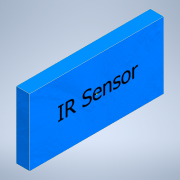
# Autodesk Inventor part: IR Sensor
Saved by Autodesk Inventor 2022.2 (Build 262287000, 287)
## iProperties
Created: 2022-02-24
Part Number: IR Sensor
Material: PVC-Piping
Document SubType Name: Modeling
Designer: PRASHANTH
Density: 1.4 g/cm^3
Appearance: Weld - Brass
Author: PRASHANTH
Autodesk Inventor part; units mm, degrees
ref_plane "YZ Plane" through (0, 0, 0) normal (1, 0, 0) x (0, 1, 0)
ref_plane "XZ Plane" through (0, 0, 0) normal (0, 1, 0) x (-1, 0, 0)
ref_plane "XY Plane" through (0, 0, 0) normal (0, 0, 1) x (1, 0, 0)
sketch "Sketch1" plane through (0, 0, 0) normal (1, 0, 0) x (0, 1, 0)
  line L0 (-7.5, 15) -> (7.5, 15)
  line L1 (7.5, 15) -> (7.5, -15)
  line L2 (7.5, -15) -> (-7.5, -15)
  line L3 (-7.5, -15) -> (-7.5, 15)
  line L4 (-7.5, 15) -> (7.5, -15) construction
  line L5 (7.5, 15) -> (-7.5, -15) construction
  point P0 (0, 0)
  dimension "d0" = 15
  dimension "d1" = 30
  constraints: 12 end point, 2 midpoint, 2 parallel, 1 horizontal, 1 perpendicular
  measures "d0" distance of L1.end L2.end
  measures "d1" distance of L0.end L1.end
extrude "Extrusion1" add sketch "Sketch1" along normal blind 3
sketch "Sketch2" plane through (3, 0, 0) normal (1, 0, 0) x (0, 0, -1)
  line L0 (-8.8041, 1.9151) -> (9.2023, 1.9151) construction
  line L1 (9.2023, 1.9151) -> (9.2023, -1.2514) construction
  line L2 (9.2023, -1.2514) -> (-8.8041, -1.2514) construction
  line L3 (-8.8041, -1.2514) -> (-8.8041, 1.9151) construction
  point P0 (0, 0)
  constraints: 2 other
body "Solid1"
